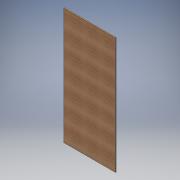
# Autodesk Inventor part: table
Saved by Autodesk Inventor 2016 (Build 200138000, 138)
## iProperties
Created: 2017-09-07
Part Number: table
Material: Wood (Birch)
Document SubType Name: Modeling
Designer: Davide
Density: 0.55 g/cm^3
Appearance: Birch - Natural Polished
Author: Davide
Autodesk Inventor part; units mm, degrees
ref_plane "YZ Plane" through (0, 0, 0) normal (1, 0, 0) x (0, 1, 0)
ref_plane "XZ Plane" through (0, 0, 0) normal (0, 1, 0) x (-1, 0, 0)
ref_plane "XY Plane" through (0, 0, 0) normal (0, 0, 1) x (1, 0, 0)
sketch "Sketch1" plane through (0, 0, 0) normal (0, 1, 0) x (-1, 0, 0)
  line L0 (259.6237, 510.3169) -> (-540.3763, 510.3169)
  line L1 (-540.3763, 510.3169) -> (-540.3763, -1289.6831)
  line L2 (-540.3763, -1289.6831) -> (259.6237, -1289.6831)
  line L3 (259.6237, -1289.6831) -> (259.6237, 510.3169)
  point P0 (0, 0)
  dimension "d0" = 1800
  dimension "d1" = 800
  constraints: 8 end point, 2 parallel, 1 horizontal, 1 perpendicular
  measures "d0" distance of L2.end L0.start
  measures "d1" distance of L1.end L2.end
extrude "Extrusion1" add sketch "Sketch1" along normal blind 15
fillet "Fillet1" radius 2 12 edges at (540.3763, 0, -389.6831) (540.3763, 7.5, -1289.6831) (540.3763, 15, -389.6831) (540.3763, 7.5, 510.3169) (140.3763, 0, 510.3169) (140.3763, 15, 510.3169) (-259.6237, 7.5, 510.3169) (-259.6237, 0, -389.6831) (-259.6237, 15, -389.6831) (-259.6237, 7.5, -1289.6831) (140.3763, 0, -1289.6831) (140.3763, 15, -1289.6831)
body "Solid1"
